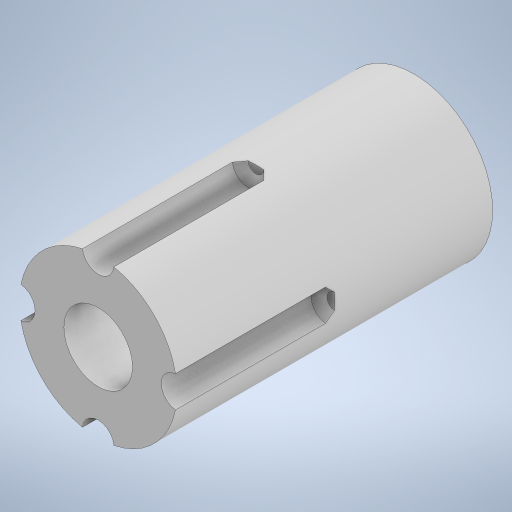
# Autodesk Inventor part: Raspberry Pi Camera v.1 Focus Tool
Saved by Autodesk Inventor 2023.2 (Build 272271000, 271)
## iProperties
Created: 2023-04-26
Part Number: Raspberry Pi Camera v.1 Focus Tool
Material: Generisch
Document SubType Name: Modeling
Designer: hangel
Density: 1 g/cm^3
Appearance: Vorgabe
Author: hangel
Autodesk Inventor part; units mm, degrees
ref_plane "YZ Plane" through (0, 0, 0) normal (1, 0, 0) x (0, 1, 0)
ref_plane "XZ Plane" through (0, 0, 0) normal (0, 1, 0) x (-1, 0, 0)
ref_plane "XY Plane" through (0, 0, 0) normal (0, 0, 1) x (1, 0, 0)
sketch "Skizze1" plane through (0, 0, 0) normal (0, 0, 1) x (1, 0, 0)
  circle A0 centre (0, 0) radius 2.675
  circle A1 centre (0, 0) radius 5
  dimension "d0" = 5.35
  dimension "d3" = 10
  constraints: 2 centre point, 2 coincident
  measures "d0" diameter of A0
  measures "d3" diameter of A1
extrude "Extrusion1" add sketch "Skizze1" along normal blind 20
sketch "Skizze2" plane through (0, 0, 0) normal (0, 0, -1) x (-1, 0, 0)
  circle A0 centre (0, 0) radius 2.675 projected
  circle A1 centre (2.675, 0) radius 0.5
  circle A2 centre (0, 2.675) radius 0.5
  circle A3 centre (-2.675, 0) radius 0.5
  circle A4 centre (0, -2.675) radius 0.5
  point P0 (0.4978, -2.6283)
  point P1 (-0.4978, -2.6283)
  point P2 (2.6283, 0.4978)
  point P3 (2.6283, -0.4978)
  point P4 (-0.4978, 2.6283)
  point P5 (0.4978, 2.6283)
  dimension "d4" = 1
  dimension "d7" = 360
  constraints: 4 centre point, 11 other
  measures "d4" diameter of A1
extrude "Extrusion2" add sketch "Skizze2" against normal blind 2 contours A0 A1 | A2 A0 | A0 A4 | A3 A0 | A0 A3 picked at (2.5116, 0.0962) picked at (0, 2.5049) picked at (0, -2.5049)
sketch "Skizze3" plane through (0, 0, 2) normal (0, 0, 1) x (1, 0, 0)
  circle A0 centre (0, 0) radius 2.675 projected
  circle A1 centre (0, 0) radius 2.175
  arc A2 (-2.6283, -0.4978) -> (-2.6283, 0.4978) centre (-2.675, 0) ccw projected
  constraints: 1 centre point, 1 coincident, 1 tangent
extrude "Extrusion3" add sketch "Skizze3" along normal up to surface (18 mm away)
sketch "Skizze4" plane through (0, 0, 20) normal (0, 0, 1) x (1, 0, 0)
  circle A0 centre (0, 0) radius 5 projected
  circle A1 centre (0, -5) radius 1
  circle A2 centre (5, 0) radius 1
  circle A3 centre (0, 5) radius 1
  circle A4 centre (-5, 0) radius 1
  point P0 (-0.995, 4.9)
  point P1 (0.995, 4.9)
  point P2 (4.9, 0.995)
  point P3 (4.9, -0.995)
  point P4 (0.995, -4.9)
  point P5 (-0.995, -4.9)
  point P6 (-4.9, -0.995)
  point P7 (-4.9, 0.995)
  dimension "d28" = 2
  dimension "d31" = 360
  constraints: 4 centre point, 11 other
  measures "d28" diameter of A1
extrude "Extrusion4" cut sketch "Skizze4" against normal blind 10 contours A0 A2 | A3 A0 | A0 A1 | A4 A0 picked at (4.6729, -0.1921) picked at (0, 4.6592) picked at (0, -4.6592) picked at (-4.6592, 0)
chamfer "Fase6" distance 0.5 angle 45 4 edges at (0, 4, 10) (4, 0, 10) (0, -4, 10) (-4, 0, 10)
